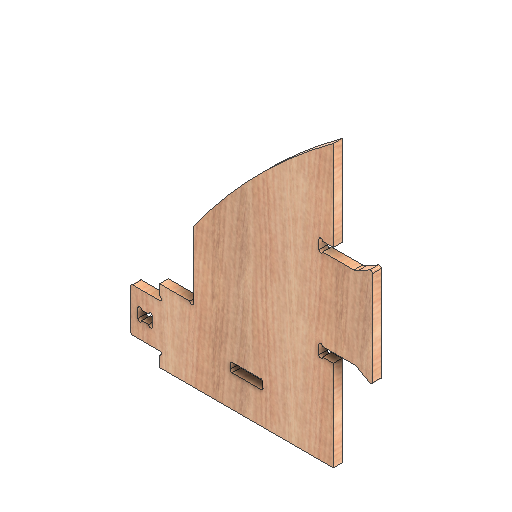
# Autodesk Inventor part: Support A
Saved by Autodesk Inventor 2021 (Build 250183000, 183)
## iProperties
Created: 2020-05-09
Part Number: Support A
Material: Wood (Birch)
Document SubType Name: Modeling
Designer: Dan Wikman
Density: 0.55 g/cm^3
Appearance: Birch - Natural Polished
Mass: 1551.32 g
Surface Area: 3577.15 cm^2
Volume: 2820.58 cm^3
Autodesk Inventor part; units mm, degrees
ref_plane "YZ Plane" through (0, 0, 0) normal (1, 0, 0) x (0, 1, 0)
ref_plane "XZ Plane" through (0, 0, 0) normal (0, 1, 0) x (-1, 0, 0)
ref_plane "XY Plane" through (0, 0, 0) normal (0, 0, 1) x (1, 0, 0)
sketch "CONTOURS" plane through (0, 0, 0) normal (0, 0, 1) x (1, 0, 0)
  line L0 (403.6989, 408.9999) -> (403.6989, 389.9999)
  arc A0 (403.6989, 389.9999) -> (411.6989, 389.9999) centre (407.6989, 389.9999) ccw
  line L1 (411.6989, 389.9999) -> (435.1989, 389.9999)
  line L2 (435.1989, 389.9999) -> (476.1797, 389.9999)
  arc A1 (476.1797, 389.9999) -> (483.6797, 392.0095) centre (476.1797, 404.9999) ccw
  line L3 (483.6797, 392.0095) -> (508.8399, 406.5358)
  arc A2 (514.8399, 403.0717) -> (508.8399, 406.5358) centre (510.8399, 403.0717) ccw
  line L4 (514.8399, 403.0717) -> (514.8399, 207.9281)
  arc A3 (508.8399, 204.464) -> (514.8399, 207.9281) centre (510.8399, 207.9281) ccw
  line L5 (508.8399, 204.464) -> (483.6797, 218.9903)
  arc A4 (483.6797, 218.9903) -> (476.1797, 220.9999) centre (476.1797, 205.9999) ccw
  line L6 (476.1797, 220.9999) -> (435.1989, 220.9999)
  line L7 (435.1989, 220.9999) -> (411.6989, 220.9999)
  arc A5 (411.6989, 220.9999) -> (403.6989, 220.9999) centre (407.6989, 220.9999) ccw
  line L8 (403.6989, 220.9999) -> (403.6989, 201.9999)
  arc A6 (403.6989, 201.9999) -> (411.6989, 201.9999) centre (407.6989, 201.9999) ccw
  line L9 (411.6989, 201.9999) -> (433.6989, 201.9999)
  line L10 (433.6989, 201.9999) -> (433.6989, 15)
  line L11 (433.6989, 15) -> (75.1989, 15)
  line L12 (75.1989, 15) -> (75.1989, 36.9214)
  arc A7 (75.1989, 36.9214) -> (75.1989, 44.9214) centre (75.1989, 40.9214) ccw
  line L13 (75.1989, 44.9214) -> (19.1989, 44.9214)
  arc A8 (15.1989, 48.9214) -> (19.1989, 44.9214) centre (19.1989, 48.9214) ccw
  line L14 (15.1989, 48.9214) -> (15.1989, 130.9214)
  arc A9 (19.1989, 134.9214) -> (15.1989, 130.9214) centre (19.1989, 130.9214) ccw
  line L15 (19.1989, 134.9214) -> (75.1989, 134.9214)
  arc A10 (75.1989, 134.9214) -> (75.1989, 142.9214) centre (75.1989, 138.9214) ccw
  line L16 (75.1989, 142.9214) -> (75.1989, 164.9196)
  line L17 (75.1989, 164.9196) -> (137.1989, 164.9196)
  arc A11 (137.1989, 164.9196) -> (145.1989, 164.9197) centre (141.1989, 164.9196) ccw
  line L18 (145.1989, 164.9197) -> (145.1989, 302.5006)
  arc A12 (433.6989, 594.9071) -> (145.1989, 302.5006) centre (1185.1989, -435.0792) ccw
  line L19 (433.6989, 594.9071) -> (433.6989, 408.9999)
  line L20 (433.6989, 408.9999) -> (411.6989, 408.9999)
  arc A13 (411.6989, 408.9999) -> (403.6989, 408.9999) centre (407.6989, 408.9999) ccw
  line L21 (614.1762, 219.9072) -> (573.1954, 219.9072)
  arc A14 (573.1954, 219.9072) -> (565.6954, 217.8975) centre (573.1954, 204.9072) ccw
  line L22 (565.6954, 217.8975) -> (540.5352, 203.3713)
  arc A15 (534.5352, 206.8354) -> (540.5352, 203.3713) centre (538.5352, 206.8354) ccw
  line L23 (534.5352, 206.8354) -> (534.5352, 401.979)
  arc A16 (540.5352, 405.4431) -> (534.5352, 401.979) centre (538.5352, 401.979) ccw
  line L24 (540.5352, 405.4431) -> (565.6954, 390.9168)
  arc A17 (565.6954, 390.9168) -> (573.1954, 388.9072) centre (573.1954, 403.9072) ccw
  line L25 (573.1954, 388.9072) -> (614.1762, 388.9072)
  constraints: 52 end point, 36 point on circle, 18 centre point
sketch "HOLES" plane through (0, 0, 0) normal (0, 0, 1) x (1, 0, 0)
  line L0 (760.9262, 514.4857) -> (760.9262, 525.4857)
  line L1 (2011.0851, 507.3098) -> (2010.9949, 507.2646)
  line L2 (2010.9949, 507.2646) -> (2010.904, 507.2219)
  line L3 (2010.904, 507.2219) -> (2010.8124, 507.1816)
  line L4 (2010.8124, 507.1816) -> (2010.7203, 507.1438)
  line L5 (2010.7203, 507.1438) -> (2010.6278, 507.1085)
  line L6 (2010.6278, 507.1085) -> (2010.535, 507.0757)
  line L7 (2010.535, 507.0757) -> (2010.4419, 507.0453)
  line L8 (2010.4419, 507.0453) -> (2010.3486, 507.0174)
  line L9 (2010.3486, 507.0174) -> (2010.2553, 506.9919)
  line L10 (2010.2553, 506.9919) -> (2010.162, 506.9688)
  line L11 (2010.162, 506.9688) -> (2010.0688, 506.9481)
  line L12 (2010.0688, 506.9481) -> (2009.9758, 506.9298)
  line L13 (2009.9758, 506.9298) -> (2009.8831, 506.9137)
  line L14 (2009.8831, 506.9137) -> (2009.7907, 506.9)
  line L15 (2009.7907, 506.9) -> (2009.6988, 506.8885)
  line L16 (2009.6988, 506.8885) -> (2009.6074, 506.8792)
  line L17 (2009.6074, 506.8792) -> (2009.5165, 506.872)
  line L18 (2009.5165, 506.872) -> (2009.4263, 506.867)
  line L19 (2009.4263, 506.867) -> (2009.3367, 506.864)
  line L20 (2009.3367, 506.864) -> (2009.248, 506.863)
  line L21 (2009.248, 506.863) -> (2009.1592, 506.864)
  line L22 (2009.1592, 506.864) -> (2009.0696, 506.867)
  line L23 (2009.0696, 506.867) -> (2008.9794, 506.872)
  line L24 (2008.9794, 506.872) -> (2008.8885, 506.8792)
  line L25 (2008.8885, 506.8792) -> (2008.7971, 506.8885)
  line L26 (2008.7971, 506.8885) -> (2008.7052, 506.9)
  line L27 (2008.7052, 506.9) -> (2008.6128, 506.9137)
  line L28 (2008.6128, 506.9137) -> (2008.5201, 506.9298)
  line L29 (2008.5201, 506.9298) -> (2008.4271, 506.9481)
  line L30 (2008.4271, 506.9481) -> (2008.3339, 506.9688)
  line L31 (2008.3339, 506.9688) -> (2008.2406, 506.9919)
  line L32 (2008.2406, 506.9919) -> (2008.1473, 507.0174)
  line L33 (2008.1473, 507.0174) -> (2008.0541, 507.0453)
  line L34 (2008.0541, 507.0453) -> (2007.961, 507.0757)
  line L35 (2007.961, 507.0757) -> (2007.8681, 507.1085)
  line L36 (2007.8681, 507.1085) -> (2007.7756, 507.1438)
  line L37 (2007.7756, 507.1438) -> (2007.6835, 507.1816)
  line L38 (2007.6835, 507.1816) -> (2007.5919, 507.2219)
  line L39 (2007.5919, 507.2219) -> (2007.501, 507.2646)
  line L40 (2007.501, 507.2646) -> (2007.4108, 507.3098)
  line L41 (2007.4108, 507.3098) -> (2007.3214, 507.3575)
  line L42 (2007.3214, 507.3575) -> (2007.2329, 507.4076)
  line L43 (2007.2329, 507.4076) -> (2007.1455, 507.4601)
  line L44 (2007.1455, 507.4601) -> (2007.0591, 507.515)
  line L45 (2007.0591, 507.515) -> (2006.974, 507.5722)
  line L46 (2006.974, 507.5722) -> (2006.8902, 507.6318)
  line L47 (2006.8902, 507.6318) -> (2006.8077, 507.6936)
  line L48 (2006.8077, 507.6936) -> (2006.7268, 507.7576)
  line L49 (2006.7268, 507.7576) -> (2006.6474, 507.8237)
  line L50 (2006.6474, 507.8237) -> (2006.5697, 507.892)
  line L51 (2006.5697, 507.892) -> (2006.4937, 507.9623)
  line L52 (2006.4937, 507.9623) -> (2006.4195, 508.0345)
  line L53 (2006.4195, 508.0345) -> (2006.3473, 508.1087)
  line L54 (2006.3473, 508.1087) -> (2006.277, 508.1847)
  line L55 (2006.277, 508.1847) -> (2006.2087, 508.2624)
  line L56 (2006.2087, 508.2624) -> (2006.1425, 508.3418)
  line L57 (2006.1425, 508.3418) -> (2006.0785, 508.4227)
  line L58 (2006.0785, 508.4227) -> (2006.0167, 508.5052)
  line L59 (2006.0167, 508.5052) -> (2005.9572, 508.589)
  line L60 (2005.9572, 508.589) -> (2005.9, 508.6741)
  line L61 (2005.9, 508.6741) -> (2005.8451, 508.7605)
  line L62 (2005.8451, 508.7605) -> (2005.7926, 508.8479)
  line L63 (2005.7926, 508.8479) -> (2005.7425, 508.9364)
  line L64 (2005.7425, 508.9364) -> (2005.6948, 509.0258)
  line L65 (2005.6948, 509.0258) -> (2005.6496, 509.116)
  line L66 (2005.6496, 509.116) -> (2005.6069, 509.2069)
  line L67 (2005.6069, 509.2069) -> (2005.5666, 509.2985)
  line L68 (2005.5666, 509.2985) -> (2005.5288, 509.3906)
  line L69 (2005.5288, 509.3906) -> (2005.4935, 509.4831)
  line L70 (2005.4935, 509.4831) -> (2005.4607, 509.576)
  line L71 (2005.4607, 509.576) -> (2005.4303, 509.6691)
  line L72 (2005.4303, 509.6691) -> (2005.4024, 509.7623)
  line L73 (2005.4024, 509.7623) -> (2005.3769, 509.8557)
  line L74 (2005.3769, 509.8557) -> (2005.3538, 509.949)
  line L75 (2005.3538, 509.949) -> (2005.3331, 510.0421)
  line L76 (2005.3331, 510.0421) -> (2005.3147, 510.1351)
  line L77 (2005.3147, 510.1351) -> (2005.2987, 510.2278)
  line L78 (2005.2987, 510.2278) -> (2005.285, 510.3202)
  line L79 (2005.285, 510.3202) -> (2005.2735, 510.4121)
  line L80 (2005.2735, 510.4121) -> (2005.2641, 510.5036)
  line L81 (2005.2641, 510.5036) -> (2005.257, 510.5944)
  line L82 (2005.257, 510.5944) -> (2005.2519, 510.6847)
  line L83 (2005.2519, 510.6847) -> (2005.2489, 510.7742)
  line L84 (2005.2489, 510.7742) -> (2005.248, 510.863)
  line L85 (2005.248, 510.863) -> (2005.248, 529.863)
  line L86 (2007.4108, 533.4161) -> (2007.501, 533.4613)
  line L87 (1019.1762, 529.4857) -> (1019.1762, 521.4857)
  arc A0 (1019.1762, 529.4857) -> (1011.1762, 529.4857) centre (1015.1762, 529.4857) ccw
  line L88 (997.1762, 529.4857) -> (1011.1762, 529.4857)
  arc A1 (997.1762, 529.4857) -> (989.1762, 529.4857) centre (993.1762, 529.4857) ccw
  line L89 (989.1762, 521.4857) -> (989.1762, 529.4857)
  line L90 (989.1762, 510.4857) -> (989.1762, 521.4857)
  arc A2 (989.1762, 510.4857) -> (997.1762, 510.4857) centre (993.1762, 510.4857) ccw
  arc A3 (760.9262, 514.4857) -> (764.9262, 510.4857) centre (764.9262, 514.4857) ccw
  line L91 (824.9262, 510.4857) -> (764.9262, 510.4857)
  arc A4 (824.9262, 510.4857) -> (828.9262, 514.4857) centre (824.9262, 514.4857) ccw
  line L92 (828.9262, 525.4857) -> (828.9262, 514.4857)
  arc A5 (828.9262, 525.4857) -> (824.9262, 529.4857) centre (824.9262, 525.4857) ccw
  line L93 (764.9262, 529.4857) -> (824.9262, 529.4857)
  arc A6 (764.9262, 529.4857) -> (760.9262, 525.4857) centre (764.9262, 525.4857) ccw
  line L94 (2012.9671, 509.3906) -> (2012.9293, 509.2985)
  line L95 (2012.9293, 509.2985) -> (2012.8891, 509.2069)
  line L96 (2012.8891, 509.2069) -> (2012.8463, 509.116)
  line L97 (2012.8463, 509.116) -> (2012.8011, 509.0258)
  line L98 (2012.8011, 509.0258) -> (2012.7534, 508.9364)
  line L99 (2012.7534, 508.9364) -> (2012.7033, 508.8479)
  line L100 (2012.7033, 508.8479) -> (2012.6508, 508.7605)
  line L101 (2012.6508, 508.7605) -> (2012.5959, 508.6741)
  line L102 (2012.5959, 508.6741) -> (2012.5387, 508.589)
  line L103 (2012.5387, 508.589) -> (2012.4792, 508.5052)
  line L104 (2012.4792, 508.5052) -> (2012.4174, 508.4227)
  line L105 (2012.4174, 508.4227) -> (2012.3534, 508.3418)
  line L106 (2012.3534, 508.3418) -> (2012.2872, 508.2624)
  line L107 (2012.2872, 508.2624) -> (2012.2189, 508.1847)
  line L108 (2012.2189, 508.1847) -> (2012.1487, 508.1087)
  line L109 (2012.1487, 508.1087) -> (2012.0764, 508.0345)
  line L110 (2012.0764, 508.0345) -> (2012.0022, 507.9623)
  line L111 (2012.0022, 507.9623) -> (2011.9263, 507.892)
  line L112 (2011.9263, 507.892) -> (2011.8485, 507.8237)
  line L113 (2011.8485, 507.8237) -> (2011.7692, 507.7576)
  line L114 (2011.7692, 507.7576) -> (2011.6882, 507.6936)
  line L115 (2011.6882, 507.6936) -> (2011.6058, 507.6318)
  line L116 (2011.6058, 507.6318) -> (2011.5219, 507.5722)
  line L117 (2011.5219, 507.5722) -> (2011.4368, 507.515)
  line L118 (2011.4368, 507.515) -> (2011.3505, 507.4601)
  line L119 (2011.3505, 507.4601) -> (2011.263, 507.4076)
  line L120 (2011.263, 507.4076) -> (2011.1745, 507.3575)
  line L121 (2005.248, 529.863) -> (2005.2489, 529.9518)
  line L122 (2005.2489, 529.9518) -> (2005.2519, 530.0413)
  line L123 (2005.2519, 530.0413) -> (2005.257, 530.1315)
  line L124 (2005.257, 530.1315) -> (2005.2641, 530.2224)
  line L125 (2005.2641, 530.2224) -> (2005.2735, 530.3138)
  line L126 (2005.2735, 530.3138) -> (2005.285, 530.4058)
  line L127 (2005.285, 530.4058) -> (2005.2987, 530.4981)
  line L128 (2005.2987, 530.4981) -> (2005.3147, 530.5908)
  line L129 (2005.3147, 530.5908) -> (2005.3331, 530.6838)
  line L130 (2005.3331, 530.6838) -> (2005.3538, 530.777)
  line L131 (2005.3538, 530.777) -> (2005.3769, 530.8703)
  line L132 (2005.3769, 530.8703) -> (2005.4024, 530.9636)
  line L133 (2005.4024, 530.9636) -> (2005.4303, 531.0569)
  line L134 (2005.4303, 531.0569) -> (2005.4607, 531.15)
  line L135 (2005.4607, 531.15) -> (2005.4935, 531.2428)
  line L136 (2005.4935, 531.2428) -> (2005.5288, 531.3354)
  line L137 (2005.5288, 531.3354) -> (2005.5666, 531.4274)
  line L138 (2005.5666, 531.4274) -> (2005.6069, 531.519)
  line L139 (2005.6069, 531.519) -> (2005.6496, 531.6099)
  line L140 (2005.6496, 531.6099) -> (2005.6948, 531.7002)
  line L141 (2005.6948, 531.7002) -> (2005.7425, 531.7895)
  line L142 (2005.7425, 531.7895) -> (2005.7926, 531.878)
  line L143 (2005.7926, 531.878) -> (2005.8451, 531.9655)
  line L144 (2005.8451, 531.9655) -> (2005.9, 532.0518)
  line L145 (2005.9, 532.0518) -> (2005.9572, 532.1369)
  line L146 (2005.9572, 532.1369) -> (2006.0167, 532.2208)
  line L147 (2006.0167, 532.2208) -> (2006.0785, 532.3032)
  line L148 (2006.0785, 532.3032) -> (2006.1425, 532.3842)
  line L149 (2006.1425, 532.3842) -> (2006.2087, 532.4635)
  line L150 (2006.2087, 532.4635) -> (2006.277, 532.5413)
  line L151 (2006.277, 532.5413) -> (2006.3473, 532.6172)
  line L152 (2006.3473, 532.6172) -> (2006.4195, 532.6914)
  line L153 (2006.4195, 532.6914) -> (2006.4937, 532.7637)
  line L154 (2006.4937, 532.7637) -> (2006.5697, 532.834)
  line L155 (2006.5697, 532.834) -> (2006.6474, 532.9022)
  line L156 (2006.6474, 532.9022) -> (2006.7268, 532.9684)
  line L157 (2006.7268, 532.9684) -> (2006.8077, 533.0324)
  line L158 (2006.8077, 533.0324) -> (2006.8902, 533.0942)
  line L159 (2006.8902, 533.0942) -> (2006.974, 533.1537)
  line L160 (2006.974, 533.1537) -> (2007.0591, 533.211)
  line L161 (2007.0591, 533.211) -> (2007.1455, 533.2658)
  line L162 (2007.1455, 533.2658) -> (2007.2329, 533.3183)
  line L163 (2007.2329, 533.3183) -> (2007.3214, 533.3684)
  line L164 (2007.3214, 533.3684) -> (2007.4108, 533.4161)
  line L165 (1593.7939, 99.4214) -> (1593.7939, 88.4214)
  line L166 (2007.501, 533.4613) -> (2007.5919, 533.5041)
  line L167 (2007.5919, 533.5041) -> (2007.6835, 533.5443)
  line L168 (2007.6835, 533.5443) -> (2007.7756, 533.5821)
  line L169 (2007.7756, 533.5821) -> (2007.8681, 533.6174)
  line L170 (2007.8681, 533.6174) -> (2007.961, 533.6503)
  line L171 (2007.961, 533.6503) -> (2008.0541, 533.6806)
  line L172 (2008.0541, 533.6806) -> (2008.1473, 533.7086)
  line L173 (2008.1473, 533.7086) -> (2008.2406, 533.7341)
  line L174 (2008.2406, 533.7341) -> (2008.3339, 533.7571)
  line L175 (2008.3339, 533.7571) -> (2008.4271, 533.7778)
  line L176 (2008.4271, 533.7778) -> (2008.5201, 533.7962)
  line L177 (2008.5201, 533.7962) -> (2008.6128, 533.8122)
  line L178 (2008.6128, 533.8122) -> (2008.7052, 533.826)
  line L179 (2008.7052, 533.826) -> (2008.7971, 533.8375)
  line L180 (2008.7971, 533.8375) -> (2008.8885, 533.8468)
  line L181 (2008.8885, 533.8468) -> (2008.9794, 533.8539)
  line L182 (2008.9794, 533.8539) -> (2009.0696, 533.859)
  line L183 (2009.0696, 533.859) -> (2009.1592, 533.862)
  line L184 (2009.1592, 533.862) -> (2009.248, 533.863)
  line L185 (2009.248, 533.863) -> (2009.3367, 533.862)
  line L186 (2009.3367, 533.862) -> (2009.4263, 533.859)
  line L187 (2009.4263, 533.859) -> (2009.5165, 533.8539)
  line L188 (2009.5165, 533.8539) -> (2009.6074, 533.8468)
  line L189 (2009.6074, 533.8468) -> (2009.6988, 533.8375)
  line L190 (2009.6988, 533.8375) -> (2009.7907, 533.826)
  line L191 (2009.7907, 533.826) -> (2009.8831, 533.8122)
  line L192 (2009.8831, 533.8122) -> (2009.9758, 533.7962)
  line L193 (2009.9758, 533.7962) -> (2010.0688, 533.7778)
  line L194 (2010.0688, 533.7778) -> (2010.162, 533.7571)
  line L195 (2010.162, 533.7571) -> (2010.2553, 533.7341)
  line L196 (288.4489, 95.4214) -> (288.4489, 84.4214)
  arc A7 (284.4489, 80.4214) -> (288.4489, 84.4214) centre (284.4489, 84.4214) ccw
  line L197 (284.4489, 80.4214) -> (224.4489, 80.4214)
  arc A8 (220.4489, 84.4214) -> (224.4489, 80.4214) centre (224.4489, 84.4214) ccw
  line L198 (220.4489, 84.4214) -> (220.4489, 95.4214)
  arc A9 (224.4489, 99.4214) -> (220.4489, 95.4214) centre (224.4489, 95.4214) ccw
  line L199 (224.4489, 99.4214) -> (284.4489, 99.4214)
  arc A10 (288.4489, 95.4214) -> (284.4489, 99.4214) centre (284.4489, 95.4214) ccw
  arc A11 (60.1989, 99.4214) -> (52.1989, 99.4214) centre (56.1989, 99.4214) ccw
  line L200 (60.1989, 99.4214) -> (60.1989, 88.4214)
  line L201 (60.1989, 88.4214) -> (60.1989, 80.4214)
  arc A12 (52.1989, 80.4214) -> (60.1989, 80.4214) centre (56.1989, 80.4214) ccw
  line L202 (52.1989, 80.4214) -> (38.1989, 80.4214)
  arc A13 (30.1989, 80.4214) -> (38.1989, 80.4214) centre (34.1989, 80.4214) ccw
  line L203 (30.1989, 80.4214) -> (30.1989, 88.4214)
  line L204 (30.1989, 88.4214) -> (30.1989, 99.4214)
  arc A14 (38.1989, 99.4214) -> (30.1989, 99.4214) centre (34.1989, 99.4214) ccw
  line L205 (38.1989, 99.4214) -> (52.1989, 99.4214)
  line L206 (2010.2553, 533.7341) -> (2010.3486, 533.7086)
  line L207 (2010.3486, 533.7086) -> (2010.4419, 533.6806)
  line L208 (2010.4419, 533.6806) -> (2010.535, 533.6503)
  line L209 (2010.535, 533.6503) -> (2010.6278, 533.6174)
  line L210 (2010.6278, 533.6174) -> (2010.7203, 533.5821)
  line L211 (2010.7203, 533.5821) -> (2010.8124, 533.5443)
  line L212 (2010.8124, 533.5443) -> (2010.904, 533.5041)
  line L213 (2010.904, 533.5041) -> (2010.9949, 533.4613)
  line L214 (2010.9949, 533.4613) -> (2011.0851, 533.4161)
  line L215 (2011.0851, 533.4161) -> (2011.1745, 533.3684)
  line L216 (2011.1745, 533.3684) -> (2011.263, 533.3183)
  line L217 (2011.263, 533.3183) -> (2011.3505, 533.2658)
  line L218 (2011.3505, 533.2658) -> (2011.4368, 533.211)
  line L219 (2011.4368, 533.211) -> (2011.5219, 533.1537)
  line L220 (2011.5219, 533.1537) -> (2011.6058, 533.0942)
  line L221 (2011.6058, 533.0942) -> (2011.6882, 533.0324)
  line L222 (2011.6882, 533.0324) -> (2011.7692, 532.9684)
  line L223 (2011.7692, 532.9684) -> (2011.8485, 532.9022)
  line L224 (2011.8485, 532.9022) -> (2011.9263, 532.834)
  line L225 (2011.9263, 532.834) -> (2012.0022, 532.7637)
  line L226 (2012.0022, 532.7637) -> (2012.0764, 532.6914)
  line L227 (2012.0764, 532.6914) -> (2012.1487, 532.6172)
  line L228 (2012.1487, 532.6172) -> (2012.2189, 532.5413)
  line L229 (2012.2189, 532.5413) -> (2012.2872, 532.4635)
  line L230 (2012.2872, 532.4635) -> (2012.3534, 532.3842)
  line L231 (2012.3534, 532.3842) -> (2012.4174, 532.3032)
  line L232 (2012.4174, 532.3032) -> (2012.4792, 532.2208)
  line L233 (2012.4792, 532.2208) -> (2012.5387, 532.1369)
  line L234 (2012.5387, 532.1369) -> (2012.5959, 532.0518)
  line L235 (2012.5959, 532.0518) -> (2012.6508, 531.9655)
  line L236 (2012.6508, 531.9655) -> (2012.7033, 531.878)
  line L237 (2012.7033, 531.878) -> (2012.7534, 531.7895)
  line L238 (2012.7534, 531.7895) -> (2012.8011, 531.7002)
  line L239 (2012.8011, 531.7002) -> (2012.8463, 531.6099)
  line L240 (2012.8463, 531.6099) -> (2012.8891, 531.519)
  line L241 (2012.8891, 531.519) -> (2012.9293, 531.4274)
  line L242 (2012.9293, 531.4274) -> (2012.9671, 531.3354)
  line L243 (2012.9671, 531.3354) -> (2013.0024, 531.2428)
  line L244 (2013.0024, 531.2428) -> (2013.0353, 531.15)
  line L245 (2013.0353, 531.15) -> (2013.0656, 531.0569)
  line L246 (2013.0656, 531.0569) -> (2013.0936, 530.9636)
  line L247 (2013.0936, 530.9636) -> (2013.119, 530.8703)
  line L248 (2013.119, 530.8703) -> (2013.1421, 530.777)
  line L249 (2013.1421, 530.777) -> (2013.1628, 530.6838)
  line L250 (2013.1628, 530.6838) -> (2013.1812, 530.5908)
  line L251 (2013.1812, 530.5908) -> (2013.1972, 530.4981)
  line L252 (2013.1972, 530.4981) -> (2013.211, 530.4058)
  line L253 (2013.211, 530.4058) -> (2013.2225, 530.3138)
  line L254 (2013.2225, 530.3138) -> (2013.2318, 530.2224)
  line L255 (2013.2318, 530.2224) -> (2013.2389, 530.1315)
  line L256 (2013.2389, 530.1315) -> (2013.244, 530.0413)
  line L257 (2013.244, 530.0413) -> (2013.247, 529.9518)
  line L258 (2013.247, 529.9518) -> (2013.248, 529.863)
  line L259 (2013.248, 529.863) -> (2027.248, 529.863)
  line L260 (2027.248, 529.863) -> (2027.2489, 529.9518)
  line L261 (2027.2489, 529.9518) -> (2027.2519, 530.0413)
  line L262 (2027.2519, 530.0413) -> (2027.257, 530.1315)
  line L263 (2027.257, 530.1315) -> (2027.2641, 530.2224)
  line L264 (2027.2641, 530.2224) -> (2027.2735, 530.3138)
  line L265 (2027.2735, 530.3138) -> (2027.285, 530.4058)
  line L266 (2027.285, 530.4058) -> (2027.2987, 530.4981)
  line L267 (2027.2987, 530.4981) -> (2027.3147, 530.5908)
  line L268 (2027.3147, 530.5908) -> (2027.3331, 530.6838)
  line L269 (2027.3331, 530.6838) -> (2027.3538, 530.777)
  line L270 (2027.3538, 530.777) -> (2027.3769, 530.8703)
  line L271 (2027.3769, 530.8703) -> (2027.4024, 530.9636)
  line L272 (2027.4024, 530.9636) -> (2027.4303, 531.0569)
  line L273 (2027.4303, 531.0569) -> (2027.4607, 531.15)
  line L274 (2027.4607, 531.15) -> (2027.4935, 531.2428)
  line L275 (2027.4935, 531.2428) -> (2027.5288, 531.3354)
  arc A15 (829.362, 99.4214) -> (821.362, 99.4214) centre (825.362, 99.4214) ccw
  line L276 (829.362, 99.4214) -> (829.362, 88.4214)
  line L277 (829.362, 88.4214) -> (829.362, 80.4214)
  arc A16 (821.362, 80.4214) -> (829.362, 80.4214) centre (825.362, 80.4214) ccw
  line L278 (821.362, 80.4214) -> (807.362, 80.4214)
  arc A17 (799.362, 80.4214) -> (807.362, 80.4214) centre (803.362, 80.4214) ccw
  line L279 (799.362, 80.4214) -> (799.362, 88.4214)
  line L280 (799.362, 88.4214) -> (799.362, 99.4214)
  arc A18 (807.362, 99.4214) -> (799.362, 99.4214) centre (803.362, 99.4214) ccw
  line L281 (807.362, 99.4214) -> (821.362, 99.4214)
  line L282 (1057.612, 95.4214) -> (1057.612, 84.4214)
  arc A19 (1053.612, 80.4214) -> (1057.612, 84.4214) centre (1053.612, 84.4214) ccw
  line L283 (1053.612, 80.4214) -> (993.612, 80.4214)
  arc A20 (989.612, 84.4214) -> (993.612, 80.4214) centre (993.612, 84.4214) ccw
  line L284 (989.612, 84.4214) -> (989.612, 95.4214)
  arc A21 (993.612, 99.4214) -> (989.612, 95.4214) centre (993.612, 95.4214) ccw
  line L285 (993.612, 99.4214) -> (1053.612, 99.4214)
  arc A22 (1057.612, 95.4214) -> (1053.612, 99.4214) centre (1053.612, 95.4214) ccw
  line L286 (2027.5288, 531.3354) -> (2027.5666, 531.4274)
  line L287 (2027.5666, 531.4274) -> (2027.6069, 531.519)
  line L288 (2027.6069, 531.519) -> (2027.6496, 531.6099)
  line L289 (2027.6496, 531.6099) -> (2027.6948, 531.7002)
  line L290 (2027.6948, 531.7002) -> (2027.7425, 531.7895)
  line L291 (2027.7425, 531.7895) -> (2027.7926, 531.878)
  line L292 (2027.7926, 531.878) -> (2027.8451, 531.9655)
  line L293 (2027.8451, 531.9655) -> (2027.9, 532.0518)
  line L294 (2027.9, 532.0518) -> (2027.9572, 532.1369)
  line L295 (2027.9572, 532.1369) -> (2028.0167, 532.2208)
  line L296 (2028.0167, 532.2208) -> (2028.0785, 532.3032)
  line L297 (2028.0785, 532.3032) -> (2028.1425, 532.3842)
  line L298 (2028.1425, 532.3842) -> (2028.2087, 532.4635)
  line L299 (2028.2087, 532.4635) -> (2028.277, 532.5413)
  line L300 (2028.277, 532.5413) -> (2028.3473, 532.6172)
  line L301 (2028.3473, 532.6172) -> (2028.4195, 532.6914)
  line L302 (2028.4195, 532.6914) -> (2028.4937, 532.7637)
  line L303 (2028.4937, 532.7637) -> (2028.5697, 532.834)
  line L304 (2028.5697, 532.834) -> (2028.6474, 532.9022)
  line L305 (2028.6474, 532.9022) -> (2028.7268, 532.9684)
  line L306 (2028.7268, 532.9684) -> (2028.8077, 533.0324)
  line L307 (2028.8077, 533.0324) -> (2028.8902, 533.0942)
  line L308 (2028.8902, 533.0942) -> (2028.974, 533.1537)
  line L309 (2028.974, 533.1537) -> (2029.0591, 533.211)
  line L310 (2029.0591, 533.211) -> (2029.1455, 533.2658)
  line L311 (2029.1455, 533.2658) -> (2029.2329, 533.3183)
  line L312 (2029.2329, 533.3183) -> (2029.3214, 533.3684)
  line L313 (2029.3214, 533.3684) -> (2029.4108, 533.4161)
  line L314 (2029.4108, 533.4161) -> (2029.501, 533.4613)
  line L315 (2029.501, 533.4613) -> (2029.5919, 533.5041)
  line L316 (2029.5919, 533.5041) -> (2029.6835, 533.5443)
  line L317 (2029.6835, 533.5443) -> (2029.7756, 533.5821)
  line L318 (2029.7756, 533.5821) -> (2029.8681, 533.6174)
  line L319 (2029.8681, 533.6174) -> (2029.961, 533.6503)
  line L320 (2029.961, 533.6503) -> (2030.0541, 533.6806)
  arc A23 (1593.7939, 99.4214) -> (1585.7939, 99.4214) centre (1589.7939, 99.4214) ccw
  line L321 (2011.1745, 507.3575) -> (2011.0851, 507.3098)
  line L322 (1593.7939, 88.4214) -> (1593.7939, 80.4214)
  arc A24 (1585.7939, 80.4214) -> (1593.7939, 80.4214) centre (1589.7939, 80.4214) ccw
  line L323 (1585.7939, 80.4214) -> (1571.7939, 80.4214)
  arc A25 (1563.7939, 80.4214) -> (1571.7939, 80.4214) centre (1567.7939, 80.4214) ccw
  line L324 (1563.7939, 80.4214) -> (1563.7939, 88.4214)
  line L325 (1563.7939, 88.4214) -> (1563.7939, 99.4214)
  arc A26 (1571.7939, 99.4214) -> (1563.7939, 99.4214) centre (1567.7939, 99.4214) ccw
  line L326 (1571.7939, 99.4214) -> (1585.7939, 99.4214)
  line L327 (1822.0439, 95.4214) -> (1822.0439, 84.4214)
  arc A27 (1818.0439, 80.4214) -> (1822.0439, 84.4214) centre (1818.0439, 84.4214) ccw
  line L328 (1818.0439, 80.4214) -> (1758.0439, 80.4214)
  arc A28 (1754.0439, 84.4214) -> (1758.0439, 80.4214) centre (1758.0439, 84.4214) ccw
  line L329 (1754.0439, 84.4214) -> (1754.0439, 95.4214)
  arc A29 (1758.0439, 99.4214) -> (1754.0439, 95.4214) centre (1758.0439, 95.4214) ccw
  line L330 (1758.0439, 99.4214) -> (1818.0439, 99.4214)
  arc A30 (1822.0439, 95.4214) -> (1818.0439, 99.4214) centre (1818.0439, 95.4214) ccw
  line L331 (2030.0541, 533.6806) -> (2030.1473, 533.7086)
  line L332 (2030.1473, 533.7086) -> (2030.2406, 533.7341)
  line L333 (2030.2406, 533.7341) -> (2030.3339, 533.7571)
  line L334 (2030.3339, 533.7571) -> (2030.4271, 533.7778)
  line L335 (2030.4271, 533.7778) -> (2030.5201, 533.7962)
  line L336 (2030.5201, 533.7962) -> (2030.6128, 533.8122)
  line L337 (2030.6128, 533.8122) -> (2030.7052, 533.826)
  line L338 (2030.7052, 533.826) -> (2030.7971, 533.8375)
  line L339 (2030.7971, 533.8375) -> (2030.8885, 533.8468)
  line L340 (2030.8885, 533.8468) -> (2030.9794, 533.8539)
  line L341 (2030.9794, 533.8539) -> (2031.0696, 533.859)
  line L342 (2031.0696, 533.859) -> (2031.1592, 533.862)
  line L343 (2031.1592, 533.862) -> (2031.248, 533.863)
  line L344 (2031.248, 533.863) -> (2031.3367, 533.862)
  line L345 (2031.3367, 533.862) -> (2031.4263, 533.859)
  line L346 (2031.4263, 533.859) -> (2031.5165, 533.8539)
  line L347 (2031.5165, 533.8539) -> (2031.6074, 533.8468)
  line L348 (2031.6074, 533.8468) -> (2031.6988, 533.8375)
  line L349 (2031.6988, 533.8375) -> (2031.7907, 533.826)
  line L350 (2031.7907, 533.826) -> (2031.8831, 533.8122)
  line L351 (2031.8831, 533.8122) -> (2031.9758, 533.7962)
  line L352 (2031.9758, 533.7962) -> (2032.0688, 533.7778)
  line L353 (2032.0688, 533.7778) -> (2032.162, 533.7571)
  line L354 (2032.162, 533.7571) -> (2032.2553, 533.7341)
  line L355 (2032.2553, 533.7341) -> (2032.3486, 533.7086)
  line L356 (2032.3486, 533.7086) -> (2032.4419, 533.6806)
  line L357 (2032.4419, 533.6806) -> (2032.535, 533.6503)
  line L358 (2032.535, 533.6503) -> (2032.6278, 533.6174)
  line L359 (2032.6278, 533.6174) -> (2032.7203, 533.5821)
  line L360 (2032.7203, 533.5821) -> (2032.8124, 533.5443)
  line L361 (2032.8124, 533.5443) -> (2032.904, 533.5041)
  line L362 (2032.904, 533.5041) -> (2032.9949, 533.4613)
  line L363 (2032.9949, 533.4613) -> (2033.0851, 533.4161)
  line L364 (2033.0851, 533.4161) -> (2033.1745, 533.3684)
  line L365 (2033.1745, 533.3684) -> (2033.263, 533.3183)
  arc A31 (1753.6081, 510.4857) -> (1761.6081, 510.4857) centre (1757.6081, 510.4857) ccw
  line L366 (1753.6081, 510.4857) -> (1753.6081, 521.4857)
  line L367 (1753.6081, 521.4857) -> (1753.6081, 529.4857)
  arc A32 (1761.6081, 529.4857) -> (1753.6081, 529.4857) centre (1757.6081, 529.4857) ccw
  line L368 (1761.6081, 529.4857) -> (1775.6081, 529.4857)
  arc A33 (1783.6081, 529.4857) -> (1775.6081, 529.4857) centre (1779.6081, 529.4857) ccw
  line L369 (1783.6081, 529.4857) -> (1783.6081, 521.4857)
  line L370 (1783.6081, 521.4857) -> (1783.6081, 510.4857)
  arc A34 (1775.6081, 510.4857) -> (1783.6081, 510.4857) centre (1779.6081, 510.4857) ccw
  line L371 (1775.6081, 510.4857) -> (1761.6081, 510.4857)
  line L372 (1525.3581, 514.4857) -> (1525.3581, 525.4857)
  arc A35 (1529.3581, 529.4857) -> (1525.3581, 525.4857) centre (1529.3581, 525.4857) ccw
  line L373 (1529.3581, 529.4857) -> (1589.3581, 529.4857)
  arc A36 (1593.3581, 525.4857) -> (1589.3581, 529.4857) centre (1589.3581, 525.4857) ccw
  line L374 (1593.3581, 525.4857) -> (1593.3581, 514.4857)
  arc A37 (1589.3581, 510.4857) -> (1593.3581, 514.4857) centre (1589.3581, 514.4857) ccw
  line L375 (1589.3581, 510.4857) -> (1529.3581, 510.4857)
  arc A38 (1525.3581, 514.4857) -> (1529.3581, 510.4857) centre (1529.3581, 514.4857) ccw
  line L376 (2033.263, 533.3183) -> (2033.3505, 533.2658)
  line L377 (2033.3505, 533.2658) -> (2033.4368, 533.211)
  line L378 (2033.4368, 533.211) -> (2033.5219, 533.1537)
  line L379 (2033.5219, 533.1537) -> (2033.6058, 533.0942)
  line L380 (2033.6058, 533.0942) -> (2033.6882, 533.0324)
  line L381 (2033.6882, 533.0324) -> (2033.7692, 532.9684)
  line L382 (2033.7692, 532.9684) -> (2033.8485, 532.9022)
  line L383 (2033.8485, 532.9022) -> (2033.9263, 532.834)
  line L384 (2033.9263, 532.834) -> (2034.0022, 532.7637)
  line L385 (2034.0022, 532.7637) -> (2034.0764, 532.6914)
  line L386 (2034.0764, 532.6914) -> (2034.1487, 532.6172)
  line L387 (2034.1487, 532.6172) -> (2034.2189, 532.5413)
  line L388 (2034.2189, 532.5413) -> (2034.2872, 532.4635)
  line L389 (2034.2872, 532.4635) -> (2034.3534, 532.3842)
  line L390 (2034.3534, 532.3842) -> (2034.4174, 532.3032)
  line L391 (2034.4174, 532.3032) -> (2034.4792, 532.2208)
  line L392 (2034.4792, 532.2208) -> (2034.5387, 532.1369)
  line L393 (2034.5387, 532.1369) -> (2034.5959, 532.0518)
  line L394 (2034.5959, 532.0518) -> (2034.6508, 531.9655)
  line L395 (2034.6508, 531.9655) -> (2034.7033, 531.878)
  line L396 (2034.7033, 531.878) -> (2034.7534, 531.7895)
  line L397 (2034.7534, 531.7895) -> (2034.8011, 531.7002)
  line L398 (2034.8011, 531.7002) -> (2034.8463, 531.6099)
  line L399 (2034.8463, 531.6099) -> (2034.8891, 531.519)
  line L400 (2034.8891, 531.519) -> (2034.9293, 531.4274)
  line L401 (2034.9293, 531.4274) -> (2034.9671, 531.3354)
  line L402 (2034.9671, 531.3354) -> (2035.0024, 531.2428)
  line L403 (2035.0024, 531.2428) -> (2035.0353, 531.15)
  line L404 (2035.0353, 531.15) -> (2035.0656, 531.0569)
  line L405 (2035.0656, 531.0569) -> (2035.0936, 530.9636)
  line L406 (2035.0936, 530.9636) -> (2035.119, 530.8703)
  line L407 (2035.119, 530.8703) -> (2035.1421, 530.777)
  line L408 (2035.1421, 530.777) -> (2035.1628, 530.6838)
  line L409 (2035.1628, 530.6838) -> (2035.1812, 530.5908)
  line L410 (2035.1812, 530.5908) -> (2035.1972, 530.4981)
  line L411 (2035.1972, 530.4981) -> (2035.211, 530.4058)
  line L412 (2035.211, 530.4058) -> (2035.2225, 530.3138)
  line L413 (2035.2225, 530.3138) -> (2035.2318, 530.2224)
  line L414 (2035.2318, 530.2224) -> (2035.2389, 530.1315)
  line L415 (2035.2389, 530.1315) -> (2035.244, 530.0413)
  line L416 (2035.244, 530.0413) -> (2035.247, 529.9518)
  line L417 (2035.247, 529.9518) -> (2035.248, 529.863)
  line L418 (2035.248, 529.863) -> (2035.248, 510.863)
  line L419 (2035.248, 510.863) -> (2035.247, 510.7742)
  line L420 (2035.247, 510.7742) -> (2035.244, 510.6847)
  line L421 (2035.244, 510.6847) -> (2035.2389, 510.5944)
  line L422 (2035.2389, 510.5944) -> (2035.2318, 510.5036)
  arc A39 (1585.1407, 687.6054) -> (1593.1407, 687.6054) centre (1589.1407, 687.6054) ccw
  line L423 (1585.1407, 687.6054) -> (1571.1407, 687.6054)
  arc A40 (1563.1407, 687.6054) -> (1571.1407, 687.6054) centre (1567.1407, 687.6054) ccw
  line L424 (1563.1407, 687.6054) -> (1563.1407, 695.6054)
  line L425 (1563.1407, 695.6054) -> (1563.1407, 706.6054)
  arc A41 (1571.1407, 706.6054) -> (1563.1407, 706.6054) centre (1567.1407, 706.6054) ccw
  line L426 (1571.1407, 706.6054) -> (1585.1407, 706.6054)
  arc A42 (1593.1407, 706.6054) -> (1585.1407, 706.6054) centre (1589.1407, 706.6054) ccw
  line L427 (1593.1407, 706.6054) -> (1593.1407, 695.6054)
  line L428 (1593.1407, 695.6054) -> (1593.1407, 687.6054)
  arc A43 (2220.6803, 687.6054) -> (2228.6803, 687.6054) centre (2224.6803, 687.6054) ccw
  line L429 (2220.6803, 687.6054) -> (2206.6803, 687.6054)
  arc A44 (2198.6803, 687.6054) -> (2206.6803, 687.6054) centre (2202.6803, 687.6054) ccw
  line L430 (2198.6803, 687.6054) -> (2198.6803, 695.6054)
  line L431 (2198.6803, 695.6054) -> (2198.6803, 706.6054)
  arc A45 (2206.6803, 706.6054) -> (2198.6803, 706.6054) centre (2202.6803, 706.6054) ccw
  line L432 (2206.6803, 706.6054) -> (2220.6803, 706.6054)
  arc A46 (2228.6803, 706.6054) -> (2220.6803, 706.6054) centre (2224.6803, 706.6054) ccw
  line L433 (2228.6803, 706.6054) -> (2228.6803, 695.6054)
  line L434 (2228.6803, 695.6054) -> (2228.6803, 687.6054)
  line L435 (2035.2318, 510.5036) -> (2035.2225, 510.4121)
  line L436 (2035.2225, 510.4121) -> (2035.211, 510.3202)
  line L437 (2035.211, 510.3202) -> (2035.1972, 510.2278)
  line L438 (2035.1972, 510.2278) -> (2035.1812, 510.1351)
  line L439 (2035.1812, 510.1351) -> (2035.1628, 510.0421)
  line L440 (2035.1628, 510.0421) -> (2035.1421, 509.949)
  line L441 (2035.1421, 509.949) -> (2035.119, 509.8557)
  line L442 (2035.119, 509.8557) -> (2035.0936, 509.7623)
  line L443 (2035.0936, 509.7623) -> (2035.0656, 509.6691)
  line L444 (2035.0656, 509.6691) -> (2035.0353, 509.576)
  line L445 (2035.0353, 509.576) -> (2035.0024, 509.4831)
  line L446 (2035.0024, 509.4831) -> (2034.9671, 509.3906)
  line L447 (2034.9671, 509.3906) -> (2034.9293, 509.2985)
  line L448 (2034.9293, 509.2985) -> (2034.8891, 509.2069)
  line L449 (2034.8891, 509.2069) -> (2034.8463, 509.116)
  line L450 (2034.8463, 509.116) -> (2034.8011, 509.0258)
  line L451 (2034.8011, 509.0258) -> (2034.7534, 508.9364)
  line L452 (2034.7534, 508.9364) -> (2034.7033, 508.8479)
  line L453 (2034.7033, 508.8479) -> (2034.6508, 508.7605)
  line L454 (2034.6508, 508.7605) -> (2034.5959, 508.6741)
  line L455 (2034.5959, 508.6741) -> (2034.5387, 508.589)
  line L456 (2034.5387, 508.589) -> (2034.4792, 508.5052)
  line L457 (2034.4792, 508.5052) -> (2034.4174, 508.4227)
  line L458 (2034.4174, 508.4227) -> (2034.3534, 508.3418)
  line L459 (2034.3534, 508.3418) -> (2034.2872, 508.2624)
  line L460 (2034.2872, 508.2624) -> (2034.2189, 508.1847)
  line L461 (2034.2189, 508.1847) -> (2034.1487, 508.1087)
  line L462 (2034.1487, 508.1087) -> (2034.0764, 508.0345)
  line L463 (2034.0764, 508.0345) -> (2034.0022, 507.9623)
  line L464 (2034.0022, 507.9623) -> (2033.9263, 507.892)
  line L465 (2033.9263, 507.892) -> (2033.8485, 507.8237)
  line L466 (2033.8485, 507.8237) -> (2033.7692, 507.7576)
  line L467 (2033.7692, 507.7576) -> (2033.6882, 507.6936)
  line L468 (2033.6882, 507.6936) -> (2033.6058, 507.6318)
  line L469 (2033.6058, 507.6318) -> (2033.5219, 507.5722)
  line L470 (2033.5219, 507.5722) -> (2033.4368, 507.515)
  line L471 (2033.4368, 507.515) -> (2033.3505, 507.4601)
  line L472 (2033.3505, 507.4601) -> (2033.263, 507.4076)
  line L473 (2033.263, 507.4076) -> (2033.1745, 507.3575)
  line L474 (2033.1745, 507.3575) -> (2033.0851, 507.3098)
  line L475 (2033.0851, 507.3098) -> (2032.9949, 507.2646)
  line L476 (2032.9949, 507.2646) -> (2032.904, 507.2219)
  line L477 (2032.904, 507.2219) -> (2032.8124, 507.1816)
  line L478 (2032.8124, 507.1816) -> (2032.7203, 507.1438)
  line L479 (2032.7203, 507.1438) -> (2032.6278, 507.1085)
  line L480 (2032.6278, 507.1085) -> (2032.535, 507.0757)
  line L481 (2032.535, 507.0757) -> (2032.4419, 507.0453)
  line L482 (2032.4419, 507.0453) -> (2032.3486, 507.0174)
  line L483 (2032.3486, 507.0174) -> (2032.2553, 506.9919)
  line L484 (2032.2553, 506.9919) -> (2032.162, 506.9688)
  line L485 (2032.162, 506.9688) -> (2032.0688, 506.9481)
  line L486 (2032.0688, 506.9481) -> (2031.9758, 506.9298)
  line L487 (2031.9758, 506.9298) -> (2031.8831, 506.9137)
  line L488 (2031.8831, 506.9137) -> (2031.7907, 506.9)
  line L489 (2031.7907, 506.9) -> (2031.6988, 506.8885)
  line L490 (2031.6988, 506.8885) -> (2031.6074, 506.8792)
  line L491 (2031.6074, 506.8792) -> (2031.5165, 506.872)
  line L492 (2031.5165, 506.872) -> (2031.4263, 506.867)
  line L493 (2031.4263, 506.867) -> (2031.3367, 506.864)
  line L494 (2031.3367, 506.864) -> (2031.248, 506.863)
  line L495 (2031.248, 506.863) -> (2031.1592, 506.864)
  line L496 (2031.1592, 506.864) -> (2031.0696, 506.867)
  line L497 (2031.0696, 506.867) -> (2030.9794, 506.872)
  line L498 (2030.9794, 506.872) -> (2030.8885, 506.8792)
  line L499 (2030.8885, 506.8792) -> (2030.7971, 506.8885)
  line L500 (2030.7971, 506.8885) -> (2030.7052, 506.9)
  line L501 (2030.7052, 506.9) -> (2030.6128, 506.9137)
  line L502 (2030.6128, 506.9137) -> (2030.5201, 506.9298)
  line L503 (2030.5201, 506.9298) -> (2030.4271, 506.9481)
  line L504 (2030.4271, 506.9481) -> (2030.3339, 506.9688)
  line L505 (2030.3339, 506.9688) -> (2030.2406, 506.9919)
  line L506 (2030.2406, 506.9919) -> (2030.1473, 507.0174)
  line L507 (2030.1473, 507.0174) -> (2030.0541, 507.0453)
  line L508 (2030.0541, 507.0453) -> (2029.961, 507.0757)
  line L509 (2029.961, 507.0757) -> (2029.8681, 507.1085)
  line L510 (2029.8681, 507.1085) -> (2029.7756, 507.1438)
  line L511 (2029.7756, 507.1438) -> (2029.6835, 507.1816)
  line L512 (2029.6835, 507.1816) -> (2029.5919, 507.2219)
  line L513 (2029.5919, 507.2219) -> (2029.501, 507.2646)
  line L514 (2029.501, 507.2646) -> (2029.4108, 507.3098)
  line L515 (2029.4108, 507.3098) -> (2029.3214, 507.3575)
  line L516 (2029.3214, 507.3575) -> (2029.2329, 507.4076)
  line L517 (2029.2329, 507.4076) -> (2029.1455, 507.4601)
  line L518 (2029.1455, 507.4601) -> (2029.0591, 507.515)
  line L519 (2029.0591, 507.515) -> (2028.974, 507.5722)
  line L520 (2028.974, 507.5722) -> (2028.8902, 507.6318)
  line L521 (2028.8902, 507.6318) -> (2028.8077, 507.6936)
  line L522 (2028.8077, 507.6936) -> (2028.7268, 507.7576)
  line L523 (2028.7268, 507.7576) -> (2028.6474, 507.8237)
  line L524 (2028.6474, 507.8237) -> (2028.5697, 507.892)
  line L525 (2028.5697, 507.892) -> (2028.4937, 507.9623)
  line L526 (2028.4937, 507.9623) -> (2028.4195, 508.0345)
  line L527 (2028.4195, 508.0345) -> (2028.3473, 508.1087)
  line L528 (2028.3473, 508.1087) -> (2028.277, 508.1847)
  arc A47 (1377.7084, 1137.6087) -> (1369.7084, 1137.6087) centre (1373.7084, 1137.6087) ccw
  line L529 (1377.7084, 1137.6087) -> (1391.7084, 1137.6087)
  arc A48 (1399.7084, 1137.6087) -> (1391.7084, 1137.6087) centre (1395.7084, 1137.6087) ccw
  line L530 (1399.7084, 1137.6087) -> (1399.7084, 1129.6087)
  line L531 (1399.7084, 1129.6087) -> (1399.7084, 1118.6087)
  arc A49 (1391.7084, 1118.6087) -> (1399.7084, 1118.6087) centre (1395.7084, 1118.6087) ccw
  line L532 (1391.7084, 1118.6087) -> (1377.7084, 1118.6087)
  arc A50 (1369.7084, 1118.6087) -> (1377.7084, 1118.6087) centre (1373.7084, 1118.6087) ccw
  line L533 (1369.7084, 1118.6087) -> (1369.7084, 1129.6087)
  line L534 (1369.7084, 1129.6087) -> (1369.7084, 1137.6087)
  arc A51 (2013.248, 1137.6087) -> (2005.248, 1137.6087) centre (2009.248, 1137.6087) ccw
  line L535 (2013.248, 1137.6087) -> (2027.248, 1137.6087)
  arc A52 (2035.248, 1137.6087) -> (2027.248, 1137.6087) centre (2031.248, 1137.6087) ccw
  line L536 (2035.248, 1137.6087) -> (2035.248, 1129.6087)
  line L537 (2035.248, 1129.6087) -> (2035.248, 1118.6087)
  arc A53 (2027.248, 1118.6087) -> (2035.248, 1118.6087) centre (2031.248, 1118.6087) ccw
  line L538 (2027.248, 1118.6087) -> (2013.248, 1118.6087)
  arc A54 (2005.248, 1118.6087) -> (2013.248, 1118.6087) centre (2009.248, 1118.6087) ccw
  line L539 (2005.248, 1118.6087) -> (2005.248, 1129.6087)
  line L540 (2005.248, 1129.6087) -> (2005.248, 1137.6087)
  line L541 (2028.277, 508.1847) -> (2028.2087, 508.2624)
  line L542 (2028.2087, 508.2624) -> (2028.1425, 508.3418)
  line L543 (2028.1425, 508.3418) -> (2028.0785, 508.4227)
  line L544 (2028.0785, 508.4227) -> (2028.0167, 508.5052)
  line L545 (2028.0167, 508.5052) -> (2027.9572, 508.589)
  line L546 (2027.9572, 508.589) -> (2027.9, 508.6741)
  line L547 (2027.9, 508.6741) -> (2027.8451, 508.7605)
  line L548 (2027.8451, 508.7605) -> (2027.7926, 508.8479)
  line L549 (2027.7926, 508.8479) -> (2027.7425, 508.9364)
  line L550 (2027.7425, 508.9364) -> (2027.6948, 509.0258)
  line L551 (2027.6948, 509.0258) -> (2027.6496, 509.116)
  line L552 (2027.6496, 509.116) -> (2027.6069, 509.2069)
  line L553 (2027.6069, 509.2069) -> (2027.5666, 509.2985)
  line L554 (2027.5666, 509.2985) -> (2027.5288, 509.3906)
  line L555 (2027.5288, 509.3906) -> (2027.4935, 509.4831)
  line L556 (2027.4935, 509.4831) -> (2027.4607, 509.576)
  line L557 (2027.4607, 509.576) -> (2027.4303, 509.6691)
  line L558 (2027.4303, 509.6691) -> (2027.4024, 509.7623)
  line L559 (2027.4024, 509.7623) -> (2027.3769, 509.8557)
  line L560 (2027.3769, 509.8557) -> (2027.3538, 509.949)
  line L561 (2027.3538, 509.949) -> (2027.3331, 510.0421)
  line L562 (2027.3331, 510.0421) -> (2027.3147, 510.1351)
  line L563 (2027.3147, 510.1351) -> (2027.2987, 510.2278)
  line L564 (2027.2987, 510.2278) -> (2027.285, 510.3202)
  line L565 (2027.285, 510.3202) -> (2027.2735, 510.4121)
  line L566 (2027.2735, 510.4121) -> (2027.2641, 510.5036)
  line L567 (2027.2641, 510.5036) -> (2027.257, 510.5944)
  line L568 (2027.257, 510.5944) -> (2027.2519, 510.6847)
  line L569 (2027.2519, 510.6847) -> (2027.2489, 510.7742)
  line L570 (2027.2489, 510.7742) -> (2027.248, 510.863)
  line L571 (2027.248, 510.863) -> (2013.248, 510.863)
  line L572 (2013.248, 510.863) -> (2013.247, 510.7742)
  line L573 (2013.247, 510.7742) -> (2013.244, 510.6847)
  line L574 (2013.244, 510.6847) -> (2013.2389, 510.5944)
  line L575 (2013.2389, 510.5944) -> (2013.2318, 510.5036)
  line L576 (2013.2318, 510.5036) -> (2013.2225, 510.4121)
  line L577 (2013.2225, 510.4121) -> (2013.211, 510.3202)
  line L578 (2013.211, 510.3202) -> (2013.1972, 510.2278)
  line L579 (2013.1972, 510.2278) -> (2013.1812, 510.1351)
  line L580 (2013.1812, 510.1351) -> (2013.1628, 510.0421)
  line L581 (2013.1628, 510.0421) -> (2013.1421, 509.949)
  line L582 (2013.1421, 509.949) -> (2013.119, 509.8557)
  line L583 (2013.119, 509.8557) -> (2013.0936, 509.7623)
  line L584 (2013.0936, 509.7623) -> (2013.0656, 509.6691)
  line L585 (2013.0656, 509.6691) -> (2013.0353, 509.576)
  line L586 (2013.0353, 509.576) -> (2013.0024, 509.4831)
  line L587 (2013.0024, 509.4831) -> (2012.9671, 509.3906)
  line L588 (1011.1762, 510.4857) -> (997.1762, 510.4857)
  arc A55 (1011.1762, 510.4857) -> (1019.1762, 510.4857) centre (1015.1762, 510.4857) ccw
  line L589 (1019.1762, 521.4857) -> (1019.1762, 510.4857)
  dimension "d53" = 19
  dimension "d55" = 30
  dimension "d63" = 68
  dimension "d71" = 30
  dimension "d75" = 19
  constraints: 1180 end point, 112 point on circle, 56 centre point
  measures "d53" distance of L165.start L322.end
  measures "d55" distance of L324.end L165.end
  measures "d63" distance between parallel lines of L329 L327
  measures "d71" distance between parallel lines of L279 L277
  measures "d75" distance between parallel lines of L285 L283
sketch "LETTERS" plane through (0, 0, 0) normal (0, 0, 1) x (1, 0, 0)
  line L0 (278.2477, 232.5818) -> (278.2477, 243.4771)
  line L1 (270.3297, 247.149) -> (290.0784, 238.0675)
  line L2 (290.0784, 238.0675) -> (270.3297, 228.76)
  constraints: 6 end point
extrude "Extrusion1" add sketch "CONTOURS" along normal blind 18
extrude "Extrusion2" cut sketch "HOLES" along normal blind 18 contours L196 A7 L197 A8 L198 A9 L199 A10 | L200 L201 A12 L202 A13 L203 L204 A14 L205 A11
body "Solid1"
